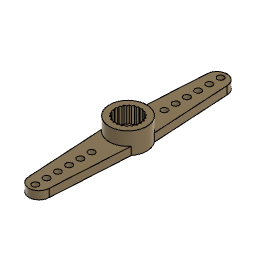
SG90_Arm_04_Custom (Autodesk Fusion 360 design; units mm, degrees)
Autodesk Fusion 360 part; units mm, degrees
sketch "スケッチ1" plane through (0, 0, 0) normal (0, 0, 1) x (1, 0, 0)
  circle A0 centre (0, 0) radius 2.45
  circle A1 centre (0, 0) radius 3.5
  line L0 (-3.5, 0) -> (3.5, 0) construction
  line L1 (0, 3.5) -> (0, -3.5) construction
  line L2 (-0.35, 2.4249) -> (0, 2.25)
  line L3 (0.35, 2.4249) -> (0, 2.25)
  line L4 (-0.35, 2.4249) -> (0.35, 2.4249) construction
  line L5 (0, 2.45) -> (0, 2.25) construction
  circle A2 centre (0, 0) radius 1.25
  line L6 (0, 3.5) -> (0, 18.5) construction
  line L7 (-2.75, 2.1651) -> (2.75, 2.1651) construction
  circle A3 centre (0, 16.6) radius 1.9
  line L8 (-1.9, 16.6) -> (1.9, 16.6) construction
  line L9 (-1.9, 16.6) -> (-2.75, 2.1651)
  line L10 (1.9, 16.6) -> (2.75, 2.1651)
  circle A4 centre (0, 17.3) radius 0.6
  circle A5 centre (0, 15.2) radius 0.6
  circle A6 centre (0, 13.1) radius 0.6
  circle A7 centre (0, 11) radius 0.6
  circle A8 centre (0, 8.9) radius 0.6
  circle A9 centre (0, 6.8) radius 0.6
  circle A10 centre (0, 0) radius 2.35
  arc A11 (1.9, 16.6) -> (-1.9, 16.6) centre (0, 16.6) ccw
  arc A12 (-1.9, -16.6) -> (1.9, -16.6) centre (0, -16.6) ccw
  line L11 (1.9, -16.6) -> (2.75, -2.1651)
  line L12 (-1.9, -16.6) -> (-2.75, -2.1651)
  circle A13 centre (0, -17.3) radius 0.6
  circle A14 centre (0, -15.2) radius 0.6
  circle A15 centre (0, -13.1) radius 0.6
  circle A16 centre (0, -11) radius 0.6
  circle A17 centre (0, -8.9) radius 0.6
  circle A18 centre (0, -6.8) radius 0.6
  dimension "d1" = 4.9
  dimension "d2" = 7
  dimension "d3" = 0.2
  dimension "d4" = 0.7
  dimension "d5" = 2.5
  dimension "d7" = 3.8
  dimension "d8" = 22
  dimension "d9" = 5.5
  dimension "d10" = 1.2
  dimension "d12" = 2.1
  dimension "d13" = 2.1
  dimension "d14" = 2.1
  dimension "d15" = 2.1
  dimension "d16" = 2.1
  dimension "d18" = 4.7
  dimension "d21" = 1.2
  constraint coincident A0.centre A1.centre
  constraint coincident A1 L0.start
  constraint coincident A1 L0.end
  constraint horizontal L0
  constraint coincident A1 L1.start
  constraint coincident A1 L1.end
  constraint perpendicular L0 L1
  constraint coincident A0 L2.start
  constraint coincident L1 L2.end
  constraint coincident A0 L3.start
  constraint horizontal L4
  constraint coincident A0 L5.start
  constraint coincident L1 L5.start
  constraint coincident A0.centre L1
  constraint concentric A1 A2
  constraint vertical L6
  constraint coincident A1 L7.start
  constraint coincident A1 L7.end
  constraint horizontal L7
  constraint coincident L6 A3.centre
  constraint coincident L6.end A3
  constraint coincident A3 L8.start
  constraint coincident A3 L8.end
  constraint perpendicular L6 L8
  constraint coincident A3.centre L8
  constraint coincident L6 A4.centre
  constraint coincident L6 A5.centre
  constraint coincident L6 A6.centre
  constraint coincident L6 A8.centre
  constraint coincident L6 A9.centre
  constraint equal A5 A6
  constraint equal A5 A7
  constraint equal A7 A8
  constraint equal A8 A9
  constraint coincident L6 A7.centre
  constraint equal A4 A5
  constraint coincident A3.centre A11.centre
  constraint symmetric L0 L7.start L12.end
  constraint symmetric L0 L7.end L11.end
  constraint symmetric L0 L8.start A12.start
  constraint symmetric L0 L8.end A12.end
  constraint symmetric L0 A4 A13
  constraint symmetric L0 A5 A14
  constraint symmetric L0 A6 A15
  constraint symmetric L0 A7 A16
  constraint symmetric L0 A8 A17
  constraint symmetric L0 A9 A18
  constraint symmetric L0 A11 A12
  constraint coincident L0 A0.centre
  measures "d1" diameter of A0
  measures "d2" diameter of A1
  measures "d3" distance of L2.end L5.start
  measures "d4" distance of L2.start L3.start
  measures "d5" diameter of A2
  measures "d7" diameter of A3
  measures "d8" distance of L1.end L6.end
  measures "d9" distance of L7.start L7.end
  measures "d10" diameter of A4
  measures "d12" distance of A4.centre A5.centre
  measures "d13" distance of A5.centre A6.centre
  measures "d14" distance of A6.centre A7.centre
  measures "d15" distance of A7.centre A8.centre
  measures "d16" distance of A8.centre A9.centre
  measures "d18" diameter of A10
  measures "d21" distance of L6.end A4.centre
extrude "押し出し1" add sketch "スケッチ1" along normal blind 1 contours A0 L2 L3 A10 | A0 L2 L3 A10 | L2 L3 A10 | L2 L3 A10 | A1
extrude "押し出し2" add sketch "スケッチ1" along normal blind 1.5 contours A1 A3 L9 L10 A5 | A1 A12 L11 L12 | A3 A5 A11
extrude "押し出し4" add sketch "スケッチ1" along normal blind 3 from surface at 1 contours A1
extrude "押し出し5" add sketch "スケッチ1" along normal up to surface (4 mm away) contours A0 L2 L3 A10 | L2 L3 A10 picked at (-0.2175, 2.4049) picked at (0, 2.3161)
pattern_circular "C パターン1" count 22 over 360 about axis through (0, 0, 1.75) along (0, 0, 1) of "押し出し5"
